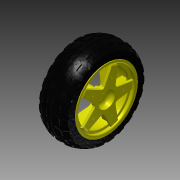
# Autodesk Inventor part: wheel
Saved by Autodesk Inventor 2015 (Build 190159000, 159)
## iProperties
Created: 2019-12-16
Part Number: wheel
Material: Generic
Document SubType Name: Modeling
Designer: Yuchofif
Density: 1 g/cm^3
Appearance: Default
Mass: 43.3033 g
Surface Area: 167.478 cm^2
Volume: 43.3033 cm^3
Author: Yuchofif
Autodesk Inventor part; units mm, degrees
sketch "Sketch1" plane through (0, 0, 0) normal (1, 0, 0) x (0, 1, 0)
  circle A0 centre (0, 0) radius 25
  circle A1 centre (0, 0) radius 22.5
  constraints: 2 centre point, 2 coincident
extrude "Extrusion1" add sketch "Sketch1" against normal blind 24.22
ref_plane "Work Plane1" through (-2.64, 0, 0) normal (1, 0, 0) x (0, 1, 0)
sketch "Sketch2" plane through (-2.64, 0, 0) normal (1, 0, 0) x (0, 1, 0)
  circle A0 centre (0, 0) radius 22.5 projected
  circle A1 centre (0, 0) radius 20.5
  constraints: 1 centre point, 1 coincident
extrude "Extrusion2" add sketch "Sketch2" against normal blind 2
sketch "Sketch3" plane through (0, 0, 0) normal (1, 0, 0) x (0, 0, -1)
  circle A0 centre (0, 0) radius 22.5 projected
  arc A1 (2.5657, 22.0512) -> (0, 22.2) centre (0, 0) ccw
  line L0 (4.6187, 8.8695) -> (2.5657, 22.0512)
  arc A2 (0, 22.2) -> (-2.5657, 22.0512) centre (0, 0) ccw
  line L1 (-4.6187, 8.8695) -> (-2.5657, 22.0512)
  arc A3 (-20.1791, 9.2544) -> (-21.1135, 6.8602) centre (0, 0) ccw
  line L2 (-7.0081, 7.1334) -> (-20.1791, 9.2544)
  arc A4 (-21.1135, 6.8602) -> (-21.7648, 4.374) centre (0, 0) ccw
  line L3 (-9.8626, -1.6518) -> (-21.7648, 4.374)
  arc A5 (-15.0371, -16.3317) -> (-13.0488, -17.9602) centre (0, 0) ccw
  line L4 (-8.9499, -4.4608) -> (-15.0371, -16.3317)
  arc A6 (-13.0488, -17.9602) -> (-10.8857, -19.3479) centre (0, 0) ccw
  line L5 (-1.4768, -9.8904) -> (-10.8857, -19.3479)
  arc A7 (10.8857, -19.3479) -> (13.0488, -17.9602) centre (0, 0) ccw
  line L6 (1.4768, -9.8904) -> (10.8857, -19.3479)
  arc A8 (13.0488, -17.9602) -> (15.0371, -16.3317) centre (0, 0) ccw
  line L7 (8.9499, -4.4608) -> (15.0371, -16.3317)
  arc A9 (21.7648, 4.374) -> (21.1135, 6.8602) centre (0, 0) ccw
  line L8 (9.8626, -1.6518) -> (21.7648, 4.374)
  arc A10 (21.1135, 6.8602) -> (20.1791, 9.2544) centre (0, 0) ccw
  line L9 (7.0081, 7.1334) -> (20.1791, 9.2544)
  line L10 (4.6187, 8.8695) -> (4.6336, 8.7768)
  line L11 (-4.6187, 8.8695) -> (-4.6336, 8.7768)
  line L12 (8.9499, -4.4608) -> (8.9075, -4.377)
  line L13 (1.4768, -9.8904) -> (1.4182, -9.8315)
  line L14 (-8.9499, -4.4608) -> (-8.912, -4.3869)
  line L15 (-9.8626, -1.6518) -> (-9.7791, -1.6946)
  line L16 (-7.0081, 7.1334) -> (-6.9261, 7.1202)
  line L17 (7.0081, 7.1334) -> (6.9261, 7.1202)
  line L18 (9.8626, -1.6518) -> (9.7885, -1.6893)
  line L19 (-1.4768, -9.8904) -> (-1.4102, -9.8242)
  arc A11 (4.6336, 8.7768) -> (6.9261, 7.1202) centre (6.6082, 9.0948) ccw
  arc A12 (-6.9261, 7.1202) -> (-4.6336, 8.7768) centre (-6.6082, 9.0948) ccw
  arc A13 (9.7885, -1.6893) -> (8.9075, -4.377) centre (10.6919, -3.4737) ccw
  arc A14 (1.4182, -9.8315) -> (-1.4102, -9.8242) centre (0.0003, -11.242) ccw
  arc A15 (-8.912, -4.3869) -> (-9.7791, -1.6946) centre (-10.6917, -3.4743) ccw
  dimension "d13" = 360
  dimension "d15" = 2
  constraints: 40 end point, 30 point on circle, 15 centre point, 10 tangent, 8 perpendicular, 4 equal radius, 2 collinear, 51 other
  measures "d15" radius of A11
extrude "Extrusion3" add sketch "Sketch3" against normal blind 2 contours L0 L10 A11 L17 L9 A10 A9 L8 L18 A13 L12 L7 A8 A7 L6 L13 A14 L19 L5 A6 A5 L4 L14 A15 L15 L3 A4 A3 L2 L16 A12 L11 L1 A2 A1
fillet "Fillet1" radius 2 5 edges at (0, 22.1628, -1.285) (0, 5.6265, -21.4751) (0, -18.6854, -11.9873) (0, -17.1747, 14.0666) (0, 8.0708, 20.681)
sketch "Sketch4" plane through (-2, 0, 0) normal (-1, 0, 0) x (0, 0, 1)
  arc A0 (21.7648, 4.374) -> (20.1791, 9.2544) centre (0, 0) ccw projected
  circle A1 centre (0, 0) radius 7.5
  circle A2 centre (0, 0) radius 6.5
  constraints: 2 centre point, 2 coincident
extrude "Extrusion4" add sketch "Sketch4" along normal blind 5 contours A1 | A2
sketch "Sketch5" plane through (0, 0, 0) normal (1, 0, 0) x (0, 0, -1)
  arc A0 (2.8863, 19.9927) -> (-2.8863, 19.9927) centre (0, 0) ccw projected
  circle A1 centre (0, 0) radius 6.5
  constraints: 1 centre point, 1 coincident
extrude "Extrusion5" cut sketch "Sketch5" against normal blind 5
fillet "Fillet2" radius 3 1 edges at (-5, 0, 6.5)
fillet "Fillet3" radius 3 1 edges at (-7, 0, -7.5)
sketch "Sketch6" plane through (-5, 0, 0) normal (1, 0, 0) x (0, 0, -1)
  circle A0 centre (0, 0) radius 3.5 projected
  circle A1 centre (0, 0) radius 2
  dimension "d28" = 4
  constraints: 1 centre point, 1 coincident
  measures "d28" diameter of A1
extrude "Extrusion6" add sketch "Sketch6" along normal blind 1.5 contours A1
fillet "Fillet4" radius 0.2 1 edges at (-3.5, 0, 2)
sketch "Sketch7" plane through (-5, 0, 0) normal (1, 0, 0) x (0, 0, -1)
  circle A0 centre (0, 2.75) radius 0.25
  circle A1 centre (2.75, 0) radius 0.25
  circle A2 centre (0, -2.75) radius 0.25
  circle A3 centre (-2.75, 0) radius 0.25
  constraints: 4 centre point
extrude "Extrusion7" add sketch "Sketch7" along normal blind 0.5
fillet "Fillet5" radius 0.2 4 edges at (-4.5, 2.75, 0.25) (-4.5, 0, -2.5) (-4.5, -2.75, 0.25) (-4.5, 0, 3)
sketch "Sketch8" plane through (0, 0, 0) normal (1, 0, 0) x (0, 0, -1)
  circle A0 centre (0, 0) radius 6.5 projected
  circle A1 centre (0, 13.5) radius 0.35
  circle A2 centre (-12.8393, 4.1717) radius 0.35
  circle A3 centre (-7.9351, -10.9217) radius 0.35
  circle A4 centre (7.9351, -10.9217) radius 0.35
  circle A5 centre (12.8393, 4.1717) radius 0.35
  dimension "d43" = 360
  constraints: 5 centre point, 11 other
extrude "Extrusion8" cut sketch "Sketch8" against normal blind 1 contours A1 | A2 | A3 | A4 | A5
fillet "Fillet6" radius 0.2 5 edges at (-1, 13.5, 0.35) (-1, 4.1717, -12.4893) (-1, -10.9217, -7.5851) (-1, -10.9217, 8.2851) (-1, 4.1717, 13.1893)
sketch "Sketch9" plane through (0, 0, 0) normal (0, 0, 1) x (1, 0, 0)
  line L0 (0, 19.9927) -> (0, 8.8695) projected
  line L1 (0, 8.8695) -> (-2, 8.8695) projected
  line L2 (-2, 22.0512) -> (-2, 8.8695) projected
  line L3 (0, 22.5) -> (0, -22.5) projected
  line L4 (-2.64, 22.5) -> (-2.64, -22.5) projected
  line L5 (-24.22, 25) -> (-24.22, -25) projected
  line L6 (0, 25) -> (0, -25) projected
  line L7 (-5, 3.5) -> (-5, -3.5) projected
  line L8 (-4, 7.5) -> (-4, -7.5) projected
  line L9 (-7, -4.5) -> (-7, 4.5) projected
  line L10 (0, -10.5717) -> (0, -11.2717) projected
  line L11 (0, 4.5217) -> (0, 3.8217) projected
  line L12 (0, 13.85) -> (0, 13.15) projected
  line L13 (0, -10.5717) -> (0, -11.2717) projected
  line L14 (0, 4.5217) -> (0, 3.8217) projected
  line L15 (0, 6.5) -> (0, -6.5) projected
  line L16 (0, 3.433) -> (0, 8.9232) projected
  line L17 (0, -1.6518) -> (0, 3.433) projected
  line L18 (0, -1.6946) -> (0, -1.6518) projected
  line L19 (0, -4.3869) -> (0, -1.6946) projected
  line L20 (0, -14.4779) -> (0, -4.3869) projected
  line L21 (0, -17.871) -> (0, -14.4779) projected
  line L22 (0, -9.8904) -> (0, -17.871) projected
  line L23 (0, -9.8242) -> (0, -9.8904) projected
  line L24 (0, -9.8315) -> (0, -9.8242) projected
  line L25 (0, -17.871) -> (0, -9.8315) projected
  line L26 (0, -14.4779) -> (0, -17.871) projected
  line L27 (0, -4.4608) -> (0, -14.4779) projected
  line L28 (0, -4.377) -> (0, -4.4608) projected
  line L29 (0, -1.6893) -> (0, -4.377) projected
  line L30 (0, 3.433) -> (0, -1.6893) projected
  line L31 (0, 8.9232) -> (0, 3.433) projected
  line L32 (0, 7.1202) -> (0, 8.9232) projected
  line L33 (0, 8.7768) -> (0, 7.1202) projected
  line L34 (0, 8.8695) -> (0, 8.7768) projected
  line L35 (0, 19.9927) -> (0, 8.8695) projected
  line L36 (0, 19.9927) -> (0, 19.9927) projected
  line L37 (0, 8.8695) -> (0, 19.9927) projected
  line L38 (0, 8.7768) -> (0, 8.8695) projected
  line L39 (0, 7.1202) -> (0, 8.7768) projected
  line L40 (0, 8.9232) -> (0, 7.1202) projected
  line L41 (0, 8.7768) -> (0, 7.1202) projected
  line L42 (0, 7.1202) -> (-2, 7.1202) projected
  line L43 (-2, 8.7768) -> (-2, 7.1202) projected
  line L44 (0, 8.7768) -> (-2, 8.7768) projected
  line L45 (-2, 7.5) -> (-4, 7.5) projected
  arc A0 (-4, 7.5) -> (-7, 4.5) centre (-4, 4.5) ccw projected
  line L46 (-2.64, 20.5) -> (-4.64, 20.5) projected
  line L47 (-4.64, -22.5) -> (-4.64, 22.5) projected
  line L48 (-4.64, 22.5) -> (-24.22, 22.5) projected
  line L49 (-2.64, 7.5) -> (-2.64, 20.5)
  line L50 (-2.64, 20.5) -> (-4.64, 20.5)
  line L51 (-4.64, 20.5) -> (-4.64, 22.5)
  line L52 (-4.64, 22.5) -> (-10.14, 22.5)
  line L53 (-10.14, 22.5) -> (-10.14, 14.5)
  line L54 (-10.14, 14.5) -> (-7, 7.9485)
  line L55 (-7, 7.9485) -> (-7, 4.5)
  arc A1 (-4, 7.5) -> (-7, 4.5) centre (-4, 4.5) ccw
  line L56 (-4, 7.5) -> (-2.64, 7.5)
  point P0 (0, 0)
  constraints: 16 end point, 4 perpendicular, 3 point on line, 3 tangent, 2 collinear, 2 point on circle, 1 centre point, 1 coincident, 1 other
extrude "Extrusion9" add sketch "Sketch9" along normal mid plane 1 contours L45 A0 L47 L46 L4 | L47 A0 L55 L54 L53 L48
fillet "Fillet7" radius 3 2 edges at (-10.14, 14.5, 0) (-7, 7.9485, 0)
pattern_circular "Circular Pattern1" count 5 over 360 about axis through (-10, 0, 0) along (1, 0, 0) of "Extrusion9", "Fillet7"
fillet "Fillet8" radius 1 1 edges at (0, -22.5, 0)
sketch "Sketch10" plane through (-7, 0, 0) normal (-1, 0, 0) x (0, 0, 1)
  arc A0 (0.7814, 4.4316) -> (0, 4.5) centre (0, 0) ccw
  arc A1 (4.2798, 1.3906) -> (0, 4.5) centre (0, 0) ccw projected
  arc A2 (0, 4.5) -> (-4.2798, 1.3906) centre (0, 0) ccw projected
  arc A3 (-4.2798, 1.3906) -> (-2.645, -3.6406) centre (0, 0) ccw projected
  arc A4 (-2.645, -3.6406) -> (2.645, -3.6406) centre (0, 0) ccw projected
  arc A5 (2.645, -3.6406) -> (4.2798, 1.3906) centre (0, 0) ccw projected
  line L0 (0.7814, 4.4316) -> (1.7073, 3.0059)
  arc A6 (0, 4.5) -> (-0.7814, 4.4316) centre (0, 0) ccw
  line L1 (-0.7814, 4.4316) -> (-1.7545, 2.9332)
  arc A7 (-3.9733, 2.1126) -> (-4.2798, 1.3906) centre (0, 0) ccw
  line L2 (-3.9733, 2.1126) -> (-2.3312, 2.5526)
  line L3 (-4.4562, 0.6263) -> (-3.3318, -0.7623)
  arc A8 (-4.2798, 1.3906) -> (-4.4562, 0.6263) centre (0, 0) ccw
  arc A9 (-3.237, -3.126) -> (-2.645, -3.6406) centre (0, 0) ccw
  line L4 (-3.237, -3.126) -> (-3.1481, -1.4283)
  line L5 (-1.9727, -4.0446) -> (-0.3046, -3.4043)
  arc A10 (-2.645, -3.6406) -> (-1.9727, -4.0446) centre (0, 0) ccw
  arc A11 (1.9727, -4.0446) -> (2.645, -3.6406) centre (0, 0) ccw
  line L6 (1.9727, -4.0446) -> (0.3856, -3.4353)
  line L7 (3.237, -3.126) -> (3.1435, -1.3417)
  arc A12 (2.645, -3.6406) -> (3.237, -3.126) centre (0, 0) ccw
  arc A13 (4.4562, 0.6263) -> (4.2798, 1.3906) centre (0, 0) ccw
  line L8 (4.4562, 0.6263) -> (3.3864, -0.6949)
  line L9 (3.9733, 2.1126) -> (2.2474, 2.5751)
  arc A14 (4.2798, 1.3906) -> (3.9733, 2.1126) centre (0, 0) ccw
  line L10 (-1.7545, 2.9332) -> (-1.9322, 2.6595)
  line L11 (-2.3312, 2.5526) -> (-1.9322, 2.6595)
  line L12 (1.7073, 3.0059) -> (1.9322, 2.6595)
  line L13 (2.2474, 2.5751) -> (1.9322, 2.6595)
  line L14 (3.3864, -0.6949) -> (3.1264, -1.0158)
  line L15 (3.1435, -1.3417) -> (3.1264, -1.0158)
  line L16 (0.3856, -3.4353) -> (0, -3.2873)
  line L17 (-0.3046, -3.4043) -> (0, -3.2873)
  line L18 (-3.3318, -0.7623) -> (-3.1264, -1.0158)
  line L19 (-3.1481, -1.4283) -> (-3.1264, -1.0158)
  dimension "d63" = 360
  constraints: 40 end point, 20 point on circle, 10 centre point, 10 collinear, 2 coincident, 49 other
extrude "Extrusion10" add sketch "Sketch10" along normal blind 3 contours L0 L12 L13 L9 A1 A5 L8 L14 L15 L7 A4 L6 L16 L17 L5 A3 L4 L19 L18 L3 A2 L2 L11 L10 L1 A0
fillet "Fillet9" radius 2 5 edges at (-8.5, 2.6595, 1.9322) (-8.5, -1.0158, 3.1264) (-8.5, -3.2873, 0) (-8.5, -1.0158, -3.1264) (-8.5, 2.6595, -1.9322)
fillet "Fillet10" radius 0.5 15 edges at (-10, 4.5, 0) (-10, 1.3906, 4.2798) (-10, 2.7746, 2.0159) (-10, 3.8675, 1.1478) (-10, -1.0598, 3.2618) (-10, 0.1035, 4.0329) (-10, -3.6406, 2.645) (-10, -3.4296, 0) (-10, -3.8035, 1.3447) (-10, -3.6406, -2.645) (-10, -1.0598, -3.2618) (-10, -2.4542, -3.2018) (-10, 1.3906, -4.2798) (-10, 2.7746, -2.0159) (-10, 2.2867, -3.3235)
sketch "Sketch11" plane through (-10, 0, 0) normal (-1, 0, 0) x (0, 0, 1)
  arc A0 (1.9417, -3.4971) -> (2.7259, -2.9273) centre (0, 0) ccw projected
  circle A1 centre (0, 0) radius 2.5
  dimension "d69" = 5
  constraints: 1 centre point, 1 coincident
  measures "d69" diameter of A1
extrude "Extrusion11" add sketch "Sketch11" along normal blind 16.8
sketch "Sketch12" plane through (-26.8, 0, 0) normal (-1, 0, 0) x (0, 0, 1)
  circle A0 centre (0, 0) radius 2.5 projected
  circle A1 centre (0, 0) radius 1.25
  dimension "d72" = 2.5
  constraints: 1 centre point, 1 coincident
  measures "d72" diameter of A1
extrude "Extrusion12" cut sketch "Sketch12" against normal blind 7 contours A1
fillet "Fillet11" radius 1.5 1 edges at (-24.22, -22.5, 0)
sketch "Sketch13" plane through (-26.8, 0, 0) normal (-1, 0, 0) x (0, 0, 1)
  circle A0 centre (0, 0) radius 2.5 projected
  circle A1 centre (0, 0) radius 2.9
  dimension "d76" = 5.8
  constraints: 1 centre point, 1 coincident
  measures "d76" diameter of A1
extrude "Extrusion13" add sketch "Sketch13" against normal blind 16.8
ref_plane "Work Plane4" through (-0.5, 0, 0) normal (1, 0, 0) x (0, 1, 0)
sketch "Sketch14" plane through (-0.5, 0, 0) normal (1, 0, 0) x (0, 1, 0)
  circle A0 centre (0, 0) radius 25 projected
  circle A1 centre (0, 0) radius 30
  constraints: 1 centre point, 1 coincident
extrude "Extrusion14" add sketch "Sketch14" against normal blind 23.22
sketch "Sketch15" plane through (0, 0, 0) normal (0, 0, 1) x (1, 0, 0)
  line L0 (-23.72, 30) -> (-23.72, -30) projected
  line L1 (-0.5, 30) -> (-0.5, -30) projected
  line L2 (-0.5, 30) -> (-23.72, 30) projected
  arc A0 (-0.5, 30) -> (-12.11, 33) centre (-11.6891, 10.6635) ccw
  arc A1 (-12.11, 33) -> (-23.72, 30) centre (-12.5309, 10.6635) ccw
  line L3 (-23.72, 30) -> (-0.5, 30)
  line L4 (-32.1607, 0) -> (5.3642, 0) projected
  point P0 (0, 0)
  constraints: 4 point on circle, 2 centre point, 2 end point, 1 collinear
revolve "Revolution1" add sketch "Sketch15" angle 360 about axis through (-10, 0, 0) along (1, 0, 0) contours A1 A0 L2
ref_plane "Work Plane5" through (0, 0, 46) normal (0, 0, 1) x (1, 0, 0)
sketch "Sketch16" plane through (0, 0, 46) normal (0, 0, 1) x (1, 0, 0)
  line L0 (-23.72, 30) -> (-23.72, -30) projected
  line L1 (-12.11, -33) -> (-12.11, 33) projected
  line L2 (-23.72, 30) -> (-23.72, -30) projected
  line L3 (-3.9, 2.5) -> (-0.5, 2.5)
  line L4 (-0.5, 2.5) -> (-0.5, -2.5)
  line L5 (-0.5, -2.5) -> (-3.9, -2.5)
  line L6 (-3.9, -2.5) -> (-3.9, 2.5)
  line L7 (-5.4, 0) -> (-5.4, -2.5)
  line L8 (-5.4, 0) -> (-5.4, 2.5)
  line L9 (-5.4, 2.5) -> (-9.2573, 4.8177)
  line L10 (-5.4, -2.5) -> (-9.2573, -0.1823)
  line L11 (-9.2573, 4.8177) -> (-9.2573, -0.1823)
  line L12 (-20.32, 2.5) -> (-23.72, 2.5)
  line L13 (-23.72, 2.5) -> (-23.72, -2.5)
  line L14 (-23.72, -2.5) -> (-20.32, -2.5)
  line L15 (-20.32, -2.5) -> (-20.32, 2.5)
  line L16 (-18.82, 0) -> (-18.82, -2.5)
  line L17 (-18.82, 0) -> (-18.82, 2.5)
  line L18 (-18.82, 2.5) -> (-14.9627, 4.8177)
  line L19 (-18.82, -2.5) -> (-14.9627, -0.1823)
  line L20 (-14.9627, 4.8177) -> (-14.9627, -0.1823)
  point P0 (0, 0)
  point P1 (-24.22, 0)
  constraints: 36 end point, 10 symmetric about line, 4 parallel, 1 collinear, 1 horizontal, 1 perpendicular
extrude "Extrusion15" add sketch "Sketch16" against normal up to surface
sketch "Sketch17" plane through (0, 0, 0) normal (0, 1, 0) x (-1, 0, 0)
  line L0 (0.5, 29.8957) -> (0.5, 29.8957) projected
  line L1 (3.9, 31.5031) -> (3.9, 31.5031) projected
  line L2 (9.2573, 32.8707) -> (9.2573, 32.5163) projected
  line L3 (5.4, 32.003) -> (5.4, 32.003) projected
  line L4 (12.11, 33) -> (12.11, -33) projected
  line L5 (23.72, 29.8957) -> (23.72, 29.8957) projected
  line L6 (20.32, 31.5031) -> (20.32, 31.5031) projected
  line L7 (14.9627, 32.5163) -> (14.9627, 32.8707) projected
  line L8 (18.82, 32.003) -> (18.82, 32.003) projected
  line L9 (12.11, 33) -> (12.11, -33) projected
  arc A0 (12.11, 33) -> (3.9, 31.6021) centre (11.6891, 10.6635) ccw projected
  arc A1 (20.32, 31.6021) -> (12.11, 33) centre (12.5309, 10.6635) ccw projected
  arc A2 (26.4386, 28.4416) -> (12.11, 34) centre (12.7658, 14.443) ccw
  arc A3 (12.11, 34) -> (-2.2186, 28.4416) centre (11.4542, 14.443) ccw
  line L10 (26.4386, 28.4416) -> (26.4386, 51.3226)
  line L11 (26.4386, 51.3226) -> (-2.2186, 51.3226)
  line L12 (-2.2186, 51.3226) -> (-2.2186, 28.4416)
  line L13 (32.966, 0) -> (-8.746, 0) projected
  point P0 (0, 0)
  constraints: 6 end point, 4 point on circle, 2 centre point, 2 parallel, 1 perpendicular, 8 other
pattern_circular "Circular Pattern2" count 23 over 360 about axis through (-10, 0, 0) along (1, 0, 0) of "Extrusion15"
revolve "Revolution2" cut sketch "Sketch17" angle 360 about axis through (-10, 0, 0) along (1, 0, 0)
ref_plane "Work Plane6" through (-12.11, 0, 0) normal (1, 0, 0) x (0, 1, 0)
sketch "Sketch18" plane through (-12.11, 0, 0) normal (1, 0, 0) x (0, 1, 0)
  circle A0 centre (0, 0) radius 32.5
  circle A1 centre (0, 0) radius 33.5
  dimension "d101" = 65
  dimension "d102" = 67
  constraints: 2 centre point, 2 coincident
  measures "d101" diameter of A0
  measures "d102" diameter of A1
extrude "Extrusion16" add sketch "Sketch18" along normal mid plane 1
body "Solid1"
